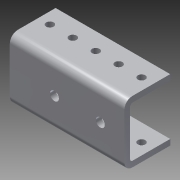
# Autodesk Inventor part: Side Mount Custom
Saved by Autodesk Inventor 2014 (Build 180170000, 170)
## iProperties
Created: 2014-01-21
Part Number: Side Mount Custom
Material: Aluminum 6061
Document SubType Name: Sheet Metal
Designer: Michael
Density: 2.71 g/cm^3
Sheet Metal Rule: Default
Appearance: Aluminum - Flat
Author: Michael
Autodesk Inventor part; units mm, degrees
ref_plane "YZ Plane" through (0, 0, 0) normal (1, 0, 0) x (0, 1, 0)
ref_plane "XZ Plane" through (0, 0, 0) normal (0, 1, 0) x (-1, 0, 0)
ref_plane "XY Plane" through (0, 0, 0) normal (0, 0, 1) x (1, 0, 0)
sketch "Sketch1" plane through (0, 0, 0) normal (0, 0, 1) x (1, 0, 0)
  line L0 (0, 0) -> (63.5, 0)
  line L1 (63.5, 0) -> (63.5, 25.4)
  line L2 (63.5, 25.4) -> (0, 25.4)
  line L3 (0, 25.4) -> (0, 0)
  circle A0 centre (24.765, 12.7) radius 2.4892
  circle A1 centre (50.165, 12.7) radius 2.4892
  dimension "d0" = 63.5
  dimension "d1" = 25.4
  dimension "d2" = 4.9784
  dimension "d5" = 25.4
  dimension "d10" = 12.7
  dimension "d11" = 24.765
  measures "d0" distance of L2.end L1.end
  measures "d1" distance of L0.end L1.end
  measures "d2" diameter of A0
  measures "d5" distance of A0.centre A1.centre
  measures "d10" distance from line of L0 A0.centre
  measures "d11" distance from line of L3 A0.centre
extrude "Plate1" add sketch "Sketch1" along normal blind 3.175
sketch "Sketch2" plane through (63.5, 26.67, -1.27) normal (0, 1, 0) x (-1, 0, 0)
  line L0 (63.5, 0) -> (0, 0)
  line L1 (0, 0) -> (0, -20.955)
  line L2 (0, -20.955) -> (63.5, -20.955)
  line L3 (63.5, -20.955) -> (63.5, 0)
  constraints: 6 end point, 1 horizontal, 1 perpendicular, 1 vertical
edge flange "Flange1" height 25.4 angle 90 thickness 3.175 bend radius 1.27 thickness toward (0, 1, 0) relief straight relief width 3.175 relief depth 1.5875 corner gap 3.175 corner form 0 edges at (31.75, 25.4, 0) (31.75, 0, 0) wall of the first edge with corners at (0, 26.67, -1.27) (63.5, 26.67, -1.27) (63.5, 26.67, -22.225) (0, 26.67, -22.225)
bend "Bend1"
corner "Corner1"
sketch "Sketch3" plane through (0, -4.445, -22.225) normal (0, -1, 0) x (1, 0, 0)
  line L0 (0, 0) -> (0, 20.955) projected
  line L1 (63.5, 0) -> (0, 0) projected
  circle A0 centre (6.35, 9.525) radius 2.0701
  circle A1 centre (19.05, 9.525) radius 2.0701
  circle A2 centre (31.75, 9.525) radius 2.0701
  circle A3 centre (44.45, 9.525) radius 2.0701
  circle A4 centre (57.15, 9.525) radius 2.0701
  point P0 (0, 22.225)
  dimension "d23" = 4.1402
  dimension "d24" = 12.7
  dimension "d25" = 6.35
  dimension "d28" = 12.7
  constraints: 5 centre point, 1 horizontal, 8 other
  measures "d23" diameter of A0
  measures "d24" vertical distance of point (0, 22.225) A0.centre
  measures "d25" distance from line of L0 A0.centre
  measures "d28" distance of A0.centre A1.centre
extrude "Extrusion1" cut sketch "Sketch3" against normal blind 50.8
equation "\"d13\" = BendReliefWidth"
equation "\"d14\" = BendReliefDepth"
equation "\"d15\" = MinimumRemnant"
equation "\"d16\" = BendRadius"
equation "\"d20\" = CornerReliefSize"
equation "\"d21\" = GapSize"
equation "\"d22\" = JacobiRadiusSize"
equation "\"BendRadius\" = Thickness"
equation "\"BendReliefWidth\" = Thickness"
equation "\"BendReliefDepth\" = 0.5 * Thickness"
equation "\"CornerReliefSize\" = 4 * Thickness"
equation "\"MinimumRemnant\" = 2 * Thickness"
equation "\"TransitionRadius\" = BendRadius"
equation "\"JacobiRadiusSize\" = BendRadius"
equation "\"GapSize\" = Thickness"
equation "\"d12\" = BendRadius"
equation "\"Thickness\" = 3.175"
body "Solid1"
